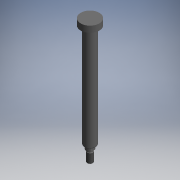
# Autodesk Inventor part: ESBF-BS-40-100-5P---(KS_0)
Saved by Autodesk Inventor 2017.3 (Build 213256000, 256)
## iProperties
Part Number: ESBF-BS-40-100-5P---(KS_0)
Material: Generic
Catalog Web Link: www.cadenas.de
Description: ESBF-(KS)-Electro-cylinder
Vendor: FESTO
Document SubType Name: Modeling
Designer: partserver
Manufacturer: FESTO
Mass: 121.055 g
Surface Area: 221.648 cm^2
Volume: 121.055 cm^3
Density: 1 g/cm^3
Appearance: PSOLRGB-128-128-128
Category: PARTsolutions
Company: FESTO
Title: ESBF-BS-40-100-5P---(KS_0)
Author: Cadenas PARTsolutions
Comments: Electro-cylinder
PSOL_IDENT_0: {$CADENAS_DATA\23d-libs\festo\parts\e\esbf\parts\esbf_ks.prj},231 {VTYP=3D},{NB=ESBF-BS-40-100-5P---
PSOL_IDENT_1: (KS_0)},{LINA=ESBF-BS-40-100-5P---(KS_0)},{NN=ESBF-(KS)},{DATE=13.05.2020 13:32:49},{GEOMDATE=17.03.
PSOL_IDENT_2: 2017 10:52:53},{VERSION=},{LINEID=50},{WBVAR=HUB,SPI,KOL,KOLE,HUBST},{WBNUMERIC=HUB,KOLE,HUBST}  {NB=
PSOL_IDENT_3: ESBF-BS-40-100-5P---(KS_0)},{LINA=ESBF-BS-40-100-5P---(KS_0)},{KT=DUMMY},{TNR=8022585},{TYP=ESBF-BS-
PSOL_IDENT_4: 40},{KDM=40},{HUB=100},{HUBMAX=1200},{SPI=5P},{KOL=-},{KOLT=},{KOLE=0},{KOLET=},{HUBST=0},{A2=0},{AM=
PSOL_IDENT_5: 24.000},{WH=29.500},{L1=14.000},{L2=144.000},{L3=18.400},{L4=14.000},{L5=3.300},{L7=9.000},{G=30.000
PSOL_IDENT_6: },{G1=30.000},{VA=7.000},{ZJ=173.500},{KK=12.000},{KKP=1.250},{MM=16.000},{D1=24.000},{D2=8.000},{D4=
PSOL_IDENT_7: 8.400},{SW1=13.000},{K1=8.000},{K1T=12.000},{X=4.000}
NB: ESBF-BS-40-100-5P---(KS_0)
NN: ESBF-(KS)
NT: Electro-cylinder
NBSYN: $TYP.-$HUB.-$SPI.$KOLT.$KOLET.---(KS_$HUBST.)
LINA: ESBF-BS-40-100-5P---(KS_0)
CATALOG: Festo
TNR: 8022585
TYP: ESBF-BS-40
KDM: 40
HUB: 100
HUBMAX: 1200
SPI: 5P
KOL: -
KOLE: 0
HUBST: 0
AM: 24
WH: 29.5
L1: 14
L2: 144
L3: 18.4
L4: 14
L5: 3.3
L7: 9
G: 30
G1: 30
VA: 7
ZJ: 173.5
KK: 12
KKP: 1.25
MM: 16
D1: 24
D2: 8
D4: 8.4
SW1: 13
K1: 8
K1T: 12
X: 4
SUPPLIER: FESTO
ARTICLENO: ESBF-BS-40-100-5P---(KS_0)
BOMINFO: ESBF-BS-40-100-5P---(KS_0)
CREATOR: CADENAS GmbH
Autodesk Inventor part; units mm, degrees
sketch "Sketch_1" plane through (0, 0, 0) normal (1, 0, 0) x (0, 1, 0)
  line L0 (0, -214) -> (0, 29.5)
  line L1 (0, 29.5) -> (7.5, 29.5)
  line L2 (7.5, 29.5) -> (8, 29)
  line L3 (8, 29) -> (8, 20.5)
  line L4 (8, 20.5) -> (11.4226, 20.5)
  line L5 (11.4226, 20.5) -> (12, 19.5)
  line L6 (12, 19.5) -> (12, -200.6667)
  line L7 (12, -200.6667) -> (20, -200.6667)
  line L8 (20, -200.6667) -> (20, -214)
  line L9 (20, -214) -> (0, -214)
  line L10 (0, -214) -> (0, 29.5)
  constraints: 22 end point
revolve "Revolution1" add sketch "Sketch_1" angle 360 about axis through (0, 0, -214) along (0, 0, -1)
sketch "Sketch_3" plane through (0, 0, 0) normal (0, 1, 0) x (-1, 0, 0)
  line L0 (9.5, 21.5) -> (9.5, 32.5)
  line L1 (9.5, 32.5) -> (-9.5, 32.5)
  line L2 (-9.5, 32.5) -> (-9.5, 21.5)
  line L3 (-9.5, 21.5) -> (-6.5, 21.5)
  line L4 (-6.5, 21.5) -> (-6.5, 29.5)
  line L5 (-6.5, 29.5) -> (6.5, 29.5)
  line L6 (6.5, 29.5) -> (6.5, 21.5)
  line L7 (6.5, 21.5) -> (9.5, 21.5)
  constraints: 16 end point
extrude "Extrusion1" cut sketch "Sketch_3" along normal mid plane 32
sketch "Sketch_2" plane through (0, 0, 0) normal (1, 0, 0) x (0, 1, 0)
  line L0 (0, 29.5) -> (0, 53.5)
  line L1 (0, 53.5) -> (5.233, 53.5)
  line L2 (5.233, 53.5) -> (6, 52.733)
  line L3 (6, 52.733) -> (6, 33.267)
  line L4 (6, 33.267) -> (5.233, 32.5)
  line L5 (5.233, 32.5) -> (5.233, 30.1)
  arc A0 (5.233, 30.1) -> (5.833, 29.5) centre (5.833, 30.1) ccw
  line L6 (5.833, 29.5) -> (0, 29.5)
  line L7 (0, 29.5) -> (0, 53.5)
  constraints: 16 end point, 2 point on circle, 1 centre point
revolve "Revolution2" add sketch "Sketch_2" angle 360 about axis through (0, 0, 29.5) along (0, 0, -1)
thread "Thread1" size "M12x1.25" class "6g" standard "ISO Metric profile" full length
ref_plane "ANBAU_XY" through (0, 0, -214) normal (0, 0, -1) x (1, 0, 0)
ref_plane "ANBAU_YZ" through (0, 0, -214) normal (1, 0, 0) x (0, -1, 0)
ref_plane "ANBAU_ZX" through (0, 0, -214) normal (0, -1, 0) x (0, 0, -1)
ref_plane "NUT_XY" through (0, 0, 37.5) normal (0, 0, -1) x (1, 0, 0)
ref_plane "NUT_YZ" through (0, 0, 37.5) normal (1, 0, 0) x (0, -1, 0)
ref_plane "NUT_ZX" through (0, 0, 37.5) normal (0, -1, 0) x (0, 0, -1)
body "Solid1"
